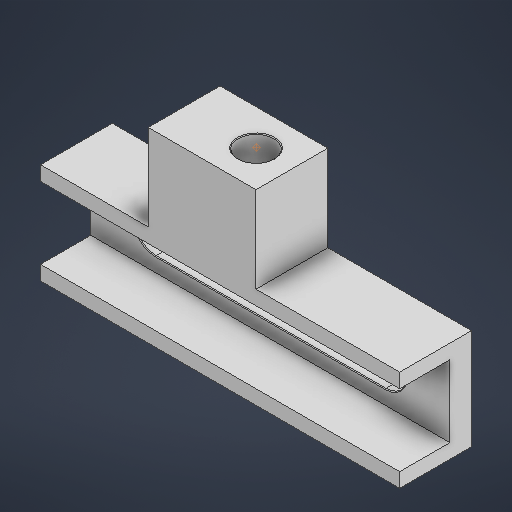
# Autodesk Inventor part: Crosshead
Saved by Autodesk Inventor 2025.4 (Build 294407000, 407)
## iProperties
Created: 2026-05-29
Part Number: Crosshead
Material: Generic
Document SubType Name: Modeling
Designer: VuQuan
Density: 1 g/cm^3
Appearance: Default
Author: VuQuan
Autodesk Inventor part; units mm, degrees
note: some values were not read from the file. Chosen so that the rebuilt part matches the saved one: direction of "Hole2".
ref_plane "YZ Plane" through (0, 0, 0) normal (1, 0, 0) x (0, 1, 0)
ref_plane "XZ Plane" through (0, 0, 0) normal (0, 1, 0) x (-1, 0, 0)
ref_plane "XY Plane" through (0, 0, 0) normal (0, 0, 1) x (1, 0, 0)
sketch "Sketch1" plane through (0, 0, 0) normal (0, 0, 1) x (1, 0, 0)
  line L0 (-25, 14) -> (-10, 14)
  line L1 (-10, 14) -> (-10, 26)
  line L2 (-10, 26) -> (5, 26)
  line L3 (5, 26) -> (5, 14)
  line L4 (5, 14) -> (25, 14)
  line L5 (25, 14) -> (25, 0)
  line L6 (25, 0) -> (-25, 0)
  line L7 (-25, 0) -> (-25, 14)
  line L8 (-16, 7) -> (16, 7) construction
  line L9 (-16, 4) -> (16, 4)
  line L10 (16, 10) -> (-16, 10)
  arc A0 (-16, 10) -> (-16, 4) centre (-16, 7) ccw
  arc A1 (16, 4) -> (16, 10) centre (16, 7) ccw
  line L11 (25, 12) -> (-25, 12)
  line L12 (-25, 2) -> (25, 2)
  point P0 (0, 0)
  point P1 (0, 0)
  point P2 (0, 7)
  point P3 (0, 26)
  point P4 (-10, 20)
  dimension "d0" = 26
  dimension "d1" = 14
  dimension "d2" = 50
  dimension "d3" = 15
  dimension "d4" = 15
  dimension "d7" = 32
  dimension "d8" = 6
  dimension "d9" = 10
  constraints: 28 end point, 8 perpendicular, 8 point on line, 4 point on circle, 4 tangent, 3 midpoint, 2 centre point, 2 horizontal, 2 vertical alignment, 1 coincident, 1 parallel, 2 other
  measures "d0" distance between parallel lines of L2 L6
  measures "d1" distance between parallel lines of L6 L0
  measures "d2" distance of L5.end L6.end
  measures "d3" distance of L0.start L0.end
  measures "d4" distance of L1.end L2.end
  measures "d7" distance of L8.start L8.end
  measures "d8" distance between parallel lines of L10 L9
  measures "d9" distance between parallel lines of L12 L11
extrude "Extrusion1" add sketch "Sketch1" along normal mid plane 10 contours L0 L1 L2 L3 L4 L5 L11 L7 | L11 L5 L12 L7 | L12 L5 L6 L7 | A0 L10 A1 L9
extrude "Extrusion2" cut sketch "Sketch1" along normal blind 5 and the other way blind 2 contours L11 L5 L12 L7
extrude "Extrusion3" cut sketch "Sketch1" along normal through all both and the other way through all contours A0 L10 A1 L9
hole "Hole1" at (0, 26, 0) direction (0, -1, 0) diameter 5 depth 10
hole "Hole2" at (-10, 20, 0) direction (1, 0, 0) diameter 3.6881 end up to surface thread size "M4.5x0.75" class "6H" standard "ISO Metric profile"
chamfer "Chamfer1" distance 0.1 angle 45 10 edges at (-10, 20, -1.8441) (0, 26, -2.5) (0, 4, -2) (19, 7, -2) (0, 10, -2) (-19, 7, -2) (0, 4, -5) (19, 7, -5) (0, 10, -5) (-19, 7, -5)
body "Solid1"
